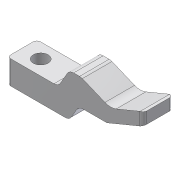
# Autodesk Inventor part: J002865
Saved by Autodesk Inventor 2012 SP2 (Build 160219200, 219)
## iProperties
Created: 2014-09-05
Material: ALUMINUM, 6061-T651
Vendor: HHMI: JFRC - ID&F
Document SubType Name: Modeling
Designer: arnoldj
Density: 2.7 g/cm^3
Mass: 17.6296 g
Surface Area: 29.9858 cm^2
Volume: 6.52949 cm^3
Description: MPS Clamp Bar
Project: P-194005
Part Number: J002865
RuleStatus: InUse
AfterDocSave0: file://Part Number Cleaner
LAB/DEPT: SVOBODA (LAB)
REQUESTING SCIENTIST: PERON, SIMON
SURFACE ROUGHNESS: 63 Ra
DESIGN DEPARTMENT: HHMI: JFRC - ID&F
SPECIAL FINISH: ANODIZE PER MIL-A-8625F, TYPE II, CLASS 2 (BLACK)
ALTERED ITEM PART NUMBER: N/A
ALTERED ITEM VENDOR: N/A
ALTERED ITEM DESCRIPTION: N/A
Revision Number: -
Autodesk Inventor part; units mm, degrees
ref_plane "YZ Plane" through (0, 0, 0) normal (1, 0, 0) x (0, 1, 0)
ref_plane "XZ Plane" through (0, 0, 0) normal (0, 1, 0) x (-1, 0, 0)
ref_plane "XY Plane" through (0, 0, 0) normal (0, 0, 1) x (1, 0, 0)
sketch "Sketch1" plane through (0, 0, 0) normal (0, 0, 1) x (1, 0, 0)
  line L0 (26.67, 7.62) -> (31.6865, 7.62)
  line L1 (31.6865, 7.62) -> (44.3865, 2.3595)
  line L2 (44.3865, 2.3595) -> (57.0865, 7.62)
  line L3 (42.7667, -3.81) -> (30.7028, -3.81)
  line L4 (57.0865, 7.62) -> (58.3565, 7.62)
  line L5 (58.3565, 7.62) -> (58.3565, 2.6475)
  line L6 (21.904, -0.635) -> (0, -0.635)
  line L7 (0, -0.635) -> (0, -10.795)
  line L8 (0, -10.795) -> (26.67, -10.795)
  line L9 (58.3565, 2.6475) -> (42.7667, -3.81)
  line L10 (26.67, 7.62) -> (21.904, -0.635)
  line L11 (26.67, -10.795) -> (30.7028, -3.81)
  point P0 (0, 0)
  dimension "d1" = 12.7
  dimension "d2" = 12.7
  dimension "d3" = 135
  dimension "d4" = 1.27
  dimension "d21" = 6.1695
  dimension "d22" = 11.43
  dimension "d45" = 5.08
  dimension "d48" = 7.62
  dimension "d49" = 0.635
  dimension "d50" = 10.16
  dimension "d56" = 26.67
  dimension "d57" = 120
  dimension "d58" = 120
  constraints: 24 end point, 3 perpendicular, 2 horizontal alignment, 2 parallel, 1 horizontal, 1 vertical alignment
  measures "d1" horizontal distance of L1.end L0.end
  measures "d2" horizontal distance of L2.end L1.end
  measures "d3" angle of L2 L1
  measures "d4" distance of L2.end L4.end
  measures "d21" distance from line of L1.end L3
  measures "d22" distance between parallel lines of L3 L0
  measures "d45" distance between parallel lines of L9 L2
  measures "d48" distance from line of point (0, 0) L0
  measures "d49" distance from line of point (0, 0) L6
  measures "d50" distance of L6.end L7.end
  measures "d56" distance from line of L0.start L7
  measures "d57" angle of L6 L10
  measures "d58" angle of L3 L11
extrude "Extrusion1" add sketch "Sketch1" along normal mid plane 12.7
sketch "Sketch3" plane through (0, -10.795, 6.35) normal (0, -1, 0) x (1, 0, 0)
  line L0 (44.3865, -12.7) -> (44.3865, 0) projected
  line L1 (26.67, 0) -> (0, 0) projected
  point P0 (0, -6.35)
  point P1 (8.001, -6.35)
  point P2 (0, -12.7)
  dimension "d26" = 36.3855
  dimension "d52" = 12.7
  dimension "d53" = 6.35
  measures "d26" distance from line of point (8.001, -6.35) L0
  measures "d52" distance of point (0, -12.7) L1.end
  measures "d53" distance from line of point (8.001, -6.35) L1
hole "Hole2" at (8.001, -10.795, 0) direction (0, 1, 0) diameter 6.3754 end through all
fillet "Fillet3" radius 6.35 1 edges at (44.3865, 2.3595, 0)
chamfer "Chamfer2" [suppressed]
fillet "Fillet5" [suppressed]
fillet "Fillet1" radius 1.5875 4 edges at (58.3565, 5.1337, 6.35) (58.3565, 5.1337, -6.35) (0, -5.715, -6.35) (0, -5.715, 6.35)
fillet "Fillet6" radius 3.175 5 edges at (21.904, -0.635, 0) (26.67, 7.62, 0) (31.6865, 7.62, 0) (26.67, -10.795, 0) (30.7028, -3.81, 0)
equation "\"d53\" = 0.5 * d52"
body "Solid1"
